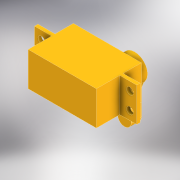
# Autodesk Inventor part: Servo
Saved by Autodesk Inventor 2021 (Build 250183000, 183)
## iProperties
Created: 2024-03-17
Part Number: Servo
Material: PLA
Document SubType Name: Modeling
Designer: Martin
Density: 1.27 g/cm^3
Appearance: PLA
Mass: 42.079 g
Surface Area: 72.9716 cm^2
Volume: 33.1331 cm^3
Author: Martin
Autodesk Inventor part; units mm, degrees
ref_plane "YZ Plane" through (0, 0, 0) normal (1, 0, 0) x (0, 1, 0)
ref_plane "XZ Plane" through (0, 0, 0) normal (0, 1, 0) x (-1, 0, 0)
sketch "Sketch1" plane through (0, 0, 0) normal (0, 1, 0) x (-1, 0, 0)
  line L0 (-20, 0) -> (20, 0)
  line L1 (20, 0) -> (20, -40.5)
  line L2 (20, -40.5) -> (-20, -40.5)
  line L3 (-20, -40.5) -> (-20, 0)
  point P0 (0, 0)
  point P1 (0, -40.5)
  dimension "d0" = 40
  dimension "d1" = 40.5
  constraints: 8 end point, 2 parallel, 1 horizontal, 1 midpoint, 1 perpendicular
  measures "d0" distance of L1.end L2.end
  measures "d1" distance of L0.end L1.end
extrude "Extrusion1" add sketch "Sketch1" along normal blind 20
sketch "Sketch2" plane through (20, 0, 0) normal (1, 0, 0) x (0, 0, -1)
  line L0 (27.7, 20) -> (29.7, 20)
  line L1 (29.7, 20) -> (29.7, 0)
  line L2 (29.7, 0) -> (27.7, 0)
  line L3 (27.7, 0) -> (27.7, 20)
  line L4 (40.5, 0) -> (40.5, 20) projected
  line L5 (0, 0) -> (0, 20) projected
  dimension "d4" = 2
  dimension "d31" = 27.7
  constraints: 8 end point, 2 parallel, 1 horizontal, 1 perpendicular
  measures "d4" distance of L1.end L2.end
  measures "d31" distance between parallel lines of L3 L5
extrude "Extrusion2" add sketch "Sketch2" along normal blind 10
sketch "Sketch3" plane through (20, 0, -29.7) normal (0, 0, -1) x (-1, 0, 0)
  circle A0 centre (-6, 15) radius 2
  line L0 (-10, 20) -> (-10, 0) projected
  line L1 (-10, 10) -> (0, 10)
  circle A1 centre (-6, 5) radius 2
  point P0 (20, 0)
  point P1 (-8, 6.7321)
  point P2 (-8, 3.2679)
  dimension "d9" = 4
  dimension "d13" = 5
  dimension "d33" = 4
  constraints: 2 centre point, 2 end point, 1 horizontal, 1 midpoint, 1 symmetric about line, 1 other
  measures "d9" diameter of A0
  measures "d13" distance from line of A0.centre L1
  measures "d33" distance from line of L0 A0.centre
extrude "Extrusion3" cut sketch "Sketch3" against normal up to next
sketch "Sketch4" plane through (20, 0, -40.5) normal (0, 0, -1) x (-1, 0, 0)
  circle A0 centre (10, 10) radius 3
  line L0 (0, 0) -> (0, 20) projected
  line L1 (0, 20) -> (40, 20) projected
  point P0 (20, 0)
  dimension "d16" = 6
  dimension "d17" = 10
  dimension "d18" = 10
  constraints: 1 centre point
  measures "d16" diameter of A0
  measures "d17" distance from line of L0 A0.centre
  measures "d18" distance from line of L1 A0.centre
extrude "Extrusion4" add sketch "Sketch4" along normal blind 6
mirror "Mirror1" about plane through (0, 0, 0) normal (1, 0, 0) of "Extrusion2", "Extrusion3"
ref_plane "Work Plane1" through (20, 0, -42.5) normal (0, 0, -1) x (-1, 0, 0)
sketch "Sketch6" plane through (20, 0, -40.5) normal (0, 0, -1) x (-1, 0, 0)
  line L0 (6, 0.4936) -> (6, -13.5)
  arc A0 (6, -13.5) -> (14, -13.5) centre (10, -13.5) ccw
  line L1 (14, -13.5) -> (14, 0.4936)
  arc A1 (15.7453, 5.1791) -> (14, 0.4936) centre (23.9461, -0.5435) ccw
  arc A2 (15.7453, 5.1791) -> (4.2547, 5.1791) centre (10, 10) ccw
  arc A3 (6, 0.4936) -> (4.2547, 5.1791) centre (-3.9461, -0.5435) ccw
  line L2 (14.2, 0.4832) -> (14.2, -13.5)
  arc A4 (5.8, -13.5) -> (14.2, -13.5) centre (10, -13.5) ccw
  line L3 (5.8, -13.5) -> (5.8, 0.4832)
  arc A5 (5.8, 0.4832) -> (4.0957, 5.0574) centre (-3.9461, -0.5435) ccw
  arc A6 (15.9043, 5.0574) -> (4.0957, 5.0574) centre (10, 10) ccw
  arc A7 (15.9043, 5.0574) -> (14.2, 0.4832) centre (23.9461, -0.5435) ccw
  circle A8 centre (10, 10) radius 3 projected
  point P0 (20, 0)
  dimension "d35" = 0.2
  constraints: 16 point on circle, 8 centre point, 8 end point, 5 other
  measures "d35" radial gap between concentric circles of A1 A7
extrude "Extrusion6" add sketch "Sketch6" along normal blind 6 contours A3 A2 A1 L1 A0 L0
sketch "Sketch7" plane through (-20, 0, 0) normal (0, 0, 1) x (1, 0, 0)
  line L0 (0, 0) -> (40, 0) projected
  line L1 (40, 0) -> (40, 20) projected
  line L2 (0, 20) -> (40, 20) projected
  line L3 (0, 0) -> (0, 20) projected
  point P0 (20, 0)
extrude "Extrusion7" cut sketch "Sketch7" against normal blind 14
body "Solid1"
